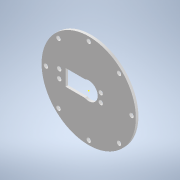
# Autodesk Inventor part: Base1
Saved by Autodesk Inventor 2021 (Build 250183000, 183)
## iProperties
Created: 2021-04-01
Part Number: Base1
Material: Genérico
Document SubType Name: Modeling
Designer: diego
Density: 1 g/cm^3
Appearance: Valor por defecto
Author: diego
Autodesk Inventor part; units mm, degrees
ref_plane "YZ Plane" through (0, 0, 0) normal (1, 0, 0) x (0, 1, 0)
ref_plane "XZ Plane" through (0, 0, 0) normal (0, 1, 0) x (-1, 0, 0)
ref_plane "XY Plane" through (0, 0, 0) normal (0, 0, 1) x (1, 0, 0)
sketch "Boceto1" plane through (0, 0, 0) normal (0, 0, 1) x (1, 0, 0)
  circle A0 centre (0, 0) radius 55
  circle A1 centre (0, 0) radius 6.5
  circle A2 centre (0, 50) radius 2.5
  circle A3 centre (-35.3553, 35.3553) radius 2.5
  circle A4 centre (-50, 0) radius 2.5
  circle A5 centre (-35.3553, -35.3553) radius 2.5
  circle A6 centre (0, -50) radius 2.5
  circle A7 centre (35.3553, -35.3553) radius 2.5
  circle A8 centre (50, 0) radius 2.5
  circle A9 centre (35.3553, 35.3553) radius 2.5
  line L0 (0, 0) -> (14, 0)
  circle A10 centre (14, 5) radius 2.5
  circle A11 centre (14, -5) radius 2.5
  circle A12 centre (-34.5, 5) radius 2.5
  circle A13 centre (-34.5, -5) radius 2.5
  dimension "d7" = 360
  constraints: 14 centre point, 2 end point, 1 coincident, 1 horizontal, 17 other
extrude "Extrusión1" add sketch "Boceto1" along normal blind 3
sketch "Boceto2" plane through (0, 0, 3) normal (0, 0, 1) x (1, 0, 0)
  point P0 (0, 0)
sketch "Boceto3" plane through (0, 0, 3) normal (0, 0, 1) x (1, 0, 0)
  arc A0 (-4.4721, -9.5) -> (-4.4721, 9.5) centre (0, 0) ccw
  line L0 (-27, 0) -> (-27, -9.5)
  line L1 (-27, -9.5) -> (-27, 9.5)
  line L2 (-27, 9.5) -> (-4.4721, 9.5)
  line L3 (-27, -9.5) -> (-4.4721, -9.5)
  constraints: 8 end point, 2 point on circle, 1 centre point, 1 coincident, 1 parallel, 1 perpendicular, 1 point on line
extrude "Extrusión2" cut sketch "Boceto3" against normal blind 3
